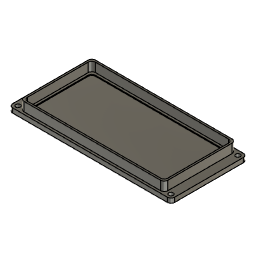
Universal case lid (Autodesk Fusion 360 design; units mm, degrees)
Autodesk Fusion 360 part; units mm, degrees
sketch "Sketch1" plane through (0, 0, 0) normal (0, 0, 1) x (1, 0, 0)
  line L0 (44.75, 21) -> (-44.75, 21)
  line L1 (-44.75, 21) -> (-44.75, -21)
  line L2 (-44.75, -21) -> (44.75, -21)
  line L3 (44.75, -21) -> (44.75, 21)
  line L4 (44.75, 21) -> (-44.75, -21) construction
  line L5 (-44.75, 21) -> (44.75, -21) construction
  circle A0 centre (-42.25, 18.5) radius 1.25
  line L6 (20, 0) -> (2.5, 0)
  circle A1 centre (-42.25, -18.5) radius 1.25
  line L7 (0, 2.5) -> (0, 20)
  circle A2 centre (42.25, -18.5) radius 1.25
  circle A3 centre (42.25, 18.5) radius 1.25
  line L8 (38.75, 18.75) -> (-38.75, 18.75)
  line L9 (-38.75, 18.75) -> (-38.75, -18.75)
  line L10 (-38.75, -18.75) -> (38.75, -18.75)
  line L11 (38.75, -18.75) -> (38.75, 18.75)
  line L12 (38.75, 18.75) -> (-38.75, -18.75) construction
  line L13 (-38.75, 18.75) -> (38.75, -18.75) construction
  line L14 (39.75, 19.75) -> (-39.75, 19.75)
  line L15 (-39.75, 19.75) -> (-39.75, -19.75)
  line L16 (-39.75, -19.75) -> (39.75, -19.75)
  line L17 (39.75, -19.75) -> (39.75, 19.75)
  line L18 (39.75, 19.75) -> (-39.75, -19.75) construction
  line L19 (-39.75, 19.75) -> (39.75, -19.75) construction
  line L20 (37.5, 17.5) -> (-37.5, 17.5)
  line L21 (-37.5, 17.5) -> (-37.5, -17.5)
  line L22 (-37.5, -17.5) -> (37.5, -17.5)
  line L23 (37.5, -17.5) -> (37.5, 17.5)
  line L24 (37.5, 17.5) -> (-37.5, -17.5) construction
  line L25 (-37.5, 17.5) -> (37.5, -17.5) construction
  dimension "d5" = 2.5
  dimension "d38" = 75
  dimension "d39" = 35
  dimension "d40" = 3.5
  dimension "d41" = 1.25
  dimension "d42" = 1.25
  dimension "d43" = 1.25
  dimension "d44" = 2.25
  dimension "d45" = 2.5
  dimension "d46" = 2.5
  dimension "d47" = 2.5
  constraint horizontal L0
  constraint perpendicular L0 L1
  constraint parallel L0 L2
  constraint parallel L1 L3
  constraint coincident L4 origin
  constraint coincident L5 origin
  constraint symmetric A0 L6 A1
  constraint symmetric A0 L7 A3
  constraint symmetric A1 L7 A2
  constraint horizontal L8
  constraint perpendicular L8 L9
  constraint parallel L8 L10
  constraint parallel L9 L11
  constraint coincident L12 origin
  constraint coincident L13 origin
  constraint horizontal L14
  constraint perpendicular L14 L15
  constraint parallel L14 L16
  constraint parallel L15 L17
  constraint coincident L18 origin
  constraint coincident L19 origin
  constraint horizontal L20
  constraint perpendicular L20 L21
  constraint parallel L20 L22
  constraint parallel L21 L23
  constraint coincident L24 origin
  constraint coincident L25 origin
  measures "d5" diameter of A0
  measures "d38" distance of L20.start L20.end
  measures "d39" distance of L20.start L22.end
  measures "d40" distance of L0 L20
  measures "d41" distance of L8 L20
  measures "d42" distance of L0 L14
  measures "d43" distance of L11 L23
  measures "d44" distance of L17 L23
  measures "d45" distance of A0.centre L15
  measures "d46" distance of L0 A0.centre
  measures "d47" distance of L3 A3.centre
extrude "Extrude1" add sketch "Sketch1" along normal blind 2.5 contours L0 L1 L2 L3 | L8 L9 L10 L11 | L14 L15 L16 L17 | L20 L21 L22 L23
extrude "Extrude7" add sketch "Sketch1" along normal blind 5 from surface at 2.5 contours L14 L15 L16 L17
extrude "Extrude8" cut sketch "Sketch1" against normal blind 0.5 from surface at 2.5 contours L20 L21 L22 L23
fillet "Fillet3" radius 2 16 edges at (-39.75, -19.75, 5) (-44.75, -21, 1.25) (-38.75, -18.75, 5) (-37.5, -17.5, 2.25) (-37.5, 17.5, 2.25) (-38.75, 18.75, 5) (-39.75, 19.75, 5) (-44.75, 21, 1.25) (39.75, 19.75, 5) (44.75, 21, 1.25) (39.75, -19.75, 5) (44.75, -21, 1.25) (37.5, -17.5, 2.25) (38.75, -18.75, 5) (38.75, 18.75, 5) (37.5, 17.5, 2.25)
equation "d3 = 2.5 mm"
equation "d42 = d41"
equation "d43 = d41"
equation "d44 = d40 - d41"
equation "d45 = d41 + 0.5 * d5"
equation "d46 = d41 + 0.5 * d5"
equation "d47 = d41 + 0.5 * d5"
equation "d48 = d3"
equation "d51 = d3"
